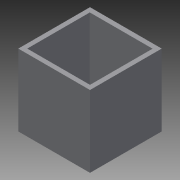
# Autodesk Inventor part: gear box
Saved by Autodesk Inventor 2015 (Build 190159000, 159)
## iProperties
Created: 2016-02-06
Part Number: gear box
Material: Generic
Document SubType Name: Modeling
Designer: Yeash
Density: 1 g/cm^3
Appearance: Default
Author: Yeash
Autodesk Inventor part; units mm, degrees
ref_plane "YZ Plane" through (0, 0, 0) normal (1, 0, 0) x (0, 1, 0)
ref_plane "XZ Plane" through (0, 0, 0) normal (0, 1, 0) x (-1, 0, 0)
ref_plane "XY Plane" through (0, 0, 0) normal (0, 0, 1) x (1, 0, 0)
sketch "Sketch1" plane through (0, 0, 0) normal (0, 1, 0) x (-1, 0, 0)
  line L0 (0, 0) -> (101.6, 0)
  line L1 (101.6, 0) -> (101.6, -101.6)
  line L2 (101.6, -101.6) -> (0, -101.6)
  line L3 (0, -101.6) -> (0, 0)
  dimension "d0" = 101.6
  dimension "d1" = 101.6
  constraints: 8 end point, 2 parallel, 1 horizontal, 1 perpendicular
  measures "d0" distance of L1.end L2.end
  measures "d1" distance of L0.end L1.end
extrude "Extrusion1" add sketch "Sketch1" along normal blind 6.35
sketch "Sketch2" plane through (0, 6.35, 0) normal (0, 1, 0) x (1, 0, 0)
  line L0 (0, 0) -> (0, 6.35)
  line L1 (0, 0) -> (0, 101.6) projected
  line L2 (-6.35, 6.35) -> (-95.25, 6.35)
  line L3 (0, 0) -> (-101.6, 0)
  line L4 (-101.6, 0) -> (0, 0) projected
  line L5 (-101.6, 0) -> (-101.6, 101.6)
  line L6 (-101.6, 101.6) -> (0, 101.6)
  line L7 (0, 0) -> (0, 101.6)
  line L8 (-101.6, 0) -> (-95.25, 0)
  line L9 (-95.25, 6.35) -> (-95.25, 94.9949)
  line L10 (-95.25, 94.9949) -> (-6.35, 94.9949)
  line L11 (-6.35, 6.35) -> (-6.35, 94.9949)
  constraints: 20 end point, 6 perpendicular, 2 point on line, 1 collinear
extrude "Extrusion2" add sketch "Sketch2" along normal blind 95.25
body "Solid1"
